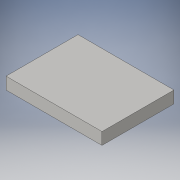
# Autodesk Inventor part: Test Part
Saved by Autodesk Inventor 2016 (Build 200138000, 138)
## iProperties
Created: 2015-12-14
Part Number: Test Part
Material: Generic
Document SubType Name: Modeling
Designer: TimB
Density: 1 g/cm^3
Appearance: Default
Author: TimB
Autodesk Inventor part; units mm, degrees
ref_plane "YZ Plane" through (0, 0, 0) normal (1, 0, 0) x (0, 1, 0)
ref_plane "XZ Plane" through (0, 0, 0) normal (0, 1, 0) x (-1, 0, 0)
ref_plane "XY Plane" through (0, 0, 0) normal (0, 0, 1) x (1, 0, 0)
sketch "Sketch1" plane through (0, 0, 0) normal (0, 1, 0) x (-1, 0, 0)
  line L0 (-101.6, 76.2) -> (101.6, 76.2)
  line L1 (101.6, 76.2) -> (101.6, -76.2)
  line L2 (101.6, -76.2) -> (-101.6, -76.2)
  line L3 (-101.6, -76.2) -> (-101.6, 76.2)
  line L4 (-101.6, 76.2) -> (101.6, -76.2) construction
  line L5 (101.6, 76.2) -> (-101.6, -76.2) construction
  point P0 (0, 0)
  dimension "d0" = 203.2
  dimension "d1" = 152.4
  constraints: 12 end point, 2 midpoint, 2 parallel, 1 horizontal, 1 perpendicular
  measures "d0" distance of L1.end L2.end
  measures "d1" distance of L0.end L1.end
extrude "Extrusion1" add sketch "Sketch1" along normal blind 25.4
body "Solid1"
